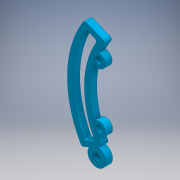
# Autodesk Inventor part: reverse gear reverse gear
Saved by Autodesk Inventor 2017 (Build 210142000, 142)
## iProperties
Created: 2018-11-14
Part Number: reverse gear reverse gear
Material: Generic
Document SubType Name: Modeling
Designer: User
Density: 1 g/cm^3
Appearance: Default
Author: User
Autodesk Inventor part; units mm, degrees
ref_plane "YZ Plane" through (0, 0, 0) normal (1, 0, 0) x (0, 1, 0)
ref_plane "XZ Plane" through (0, 0, 0) normal (0, 1, 0) x (-1, 0, 0)
ref_plane "XY Plane" through (0, 0, 0) normal (0, 0, 1) x (1, 0, 0)
sketch "Sketch1" plane through (0, 0, 0) normal (0, 1, 0) x (-1, 0, 0)
  circle A0 centre (32.4474, 13.089) radius 1.5
  circle A1 centre (32.2267, -13) radius 1.5
  arc A2 (39.8573, -23.4618) -> (38.7049, 25.3179) centre (0, 0) ccw
  line L0 (32.9955, 20.319) -> (35.5948, 21.3676)
  line L1 (29.1983, 21.483) -> (38.7049, 25.3179)
  circle A3 centre (33.2491, -24.1954) radius 1.5
  line L2 (36.25, -19.685) -> (38.5713, -20.6475)
  line L3 (35.5948, 21.3676) -> (37.6913, 22.2133)
  line L4 (33.9272, -18.7219) -> (36.25, -19.685)
  arc A4 (33.9272, -18.7219) -> (32.9955, 20.319) centre (0, 0) ccw
  arc A5 (38.5713, -20.6475) -> (37.6913, 22.2133) centre (0, 0) ccw
  arc A6 (32.4841, 16.0888) -> (29.1983, 21.483) centre (0, 0) ccw
  arc A7 (30.7875, -19.1361) -> (32.5357, -15.984) centre (0, 0) ccw
  arc A8 (34.5198, -11.0656) -> (34.5553, 10.9543) centre (0, 0) ccw
  arc A9 (32.4841, 16.0888) -> (34.5553, 10.9543) centre (32.4474, 13.089) ccw
  arc A10 (34.5198, -11.0656) -> (32.5357, -15.984) centre (32.2267, -13) ccw
  line L5 (33.2491, -20.1954) -> (30.7875, -19.1361)
  line L6 (36.643, -22.0786) -> (39.8573, -23.4618)
  arc A11 (33.2491, -20.1954) -> (36.643, -22.0786) centre (33.2491, -24.1954) ccw
  dimension "d29" = 4
  dimension "d30" = 3
  dimension "d31" = 3
  dimension "d32" = 46.25
  dimension "d33" = 43.75
  dimension "d34" = 38.75
  dimension "d35" = 36.25
  dimension "d36" = 36.25
  dimension "d37" = 0.764
  dimension "d38" = 45.253
  dimension "d39" = 0.764
  dimension "d40" = 0.3882
  dimension "d41" = 2.5
  dimension "d42" = 2.1071
  dimension "d43" = 43.1688
  dimension "d44" = 44.3514
  dimension "d45" = 2.0605
  dimension "d46" = 2.0432
  dimension "d47" = 39.4934
  dimension "d48" = 29.5173
  dimension "d49" = 9.2767
  dimension "d50" = 1.6208
  dimension "d51" = 33.4149
  dimension "d52" = 5.7959
  dimension "d53" = 4.2998
  dimension "d54" = 26.089
  constraints: 18 point on circle, 14 end point, 12 centre point, 3 coincident, 3 concentric, 3 equal radius, 3 parallel, 2 tangent
  measures "d29" radius of A11
  measures "d30" diameter of A3
  measures "d31" radius of A9
  measures "d32" radius of A2
  measures "d33" radius of A5
  measures "d34" radius of A4
  measures "d35" radius of A6
  measures "d36" radius of A8
  measures "d37" angle of L6 L2
  measures "d38" angle of L6 L3
  measures "d39" angle of L6 L4
  measures "d40" distance between parallel lines of L6 L5
  measures "d41" distance between parallel lines of L1 L3
  measures "d42" distance from line of L6.end L2
  measures "d43" distance from line of L6.end L3
  measures "d44" distance from line of L1.end L6
  measures "d45" distance from line of L6.start L2
  measures "d46" distance from line of L2.start L6
  measures "d47" distance from line of L0.end L6
  measures "d48" distance from line of A8.end L6
  measures "d49" distance from line of A8.start L6
  measures "d50" distance from line of L5.start L2
  measures "d51" distance from line of A6.start L6
  measures "d52" distance from line of point (0, 0) L6
  measures "d53" distance from line of point (0, 0) L2
  measures "d54" vertical distance of A1.centre A0.centre
extrude "Extrusion1" add sketch "Sketch1" along normal blind 3
fillet "Fillet1" radius 1 8 edges at (-29.1983, 1.5, 21.483) (-38.7049, 1.5, 25.3179) (-38.5713, 1.5, -20.6475) (-30.7875, 1.5, -19.1361) (-33.9272, 1.5, -18.7219) (-39.8573, 1.5, -23.4618) (-32.9955, 1.5, 20.319) (-37.6913, 1.5, 22.2133)
body "Solid1"
